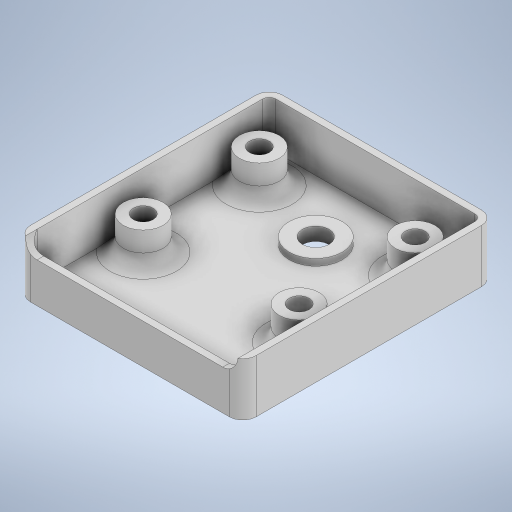
# Autodesk Inventor part: MKSMount
Saved by Autodesk Inventor 2024.2 (Build 282272000, 272)
## iProperties
Created: 2024-06-06
Part Number: MKSMount
Material: Generic
Document SubType Name: Modeling
Designer: Robin
Density: 1 g/cm^3
Appearance: Default
Author: Robin
Autodesk Inventor part; units mm, degrees
ref_plane "YZ Plane" through (0, 0, 0) normal (1, 0, 0) x (0, 1, 0)
ref_plane "XZ Plane" through (0, 0, 0) normal (0, 1, 0) x (-1, 0, 0)
ref_plane "XY Plane" through (0, 0, 0) normal (0, 0, 1) x (1, 0, 0)
sketch "Sketch1" plane through (0, 0, 0) normal (0, 1, 0) x (-1, 0, 0)
  line L0 (17, 19) -> (-17, 19)
  line L1 (-17, 19) -> (-17, -19)
  line L2 (-17, -19) -> (17, -19)
  line L3 (17, -19) -> (17, 19)
  point P0 (0, 0)
  point P1 (0, 19)
  point P2 (17, 0)
  dimension "d0" = 38
  dimension "d1" = 34
  constraints: 8 end point, 2 midpoint, 2 parallel, 1 horizontal, 1 horizontal alignment, 1 perpendicular, 1 vertical alignment
  measures "d0" distance of L2.end L0.start
  measures "d1" distance of L0.start L0.end
extrude "Extrusion1" add sketch "Sketch1" along normal blind 8
shell "Shell1" thickness 1 removed faces 1 at (5.6667, 8, 6.3333)
sketch "Sketch2" plane through (-16, 1, -18) normal (0, 1, 0) x (1, 0, 0)
  circle A0 centre (4, -23) radius 3
  circle A1 centre (4, -5.5) radius 3
  circle A2 centre (27.5, -23) radius 3
  circle A3 centre (27.5, -5.5) radius 3
  line L0 (32, -36) -> (0, -36) projected
  line L1 (0, -36) -> (0, 0) projected
  circle A4 centre (4, -23) radius 1.5
  circle A5 centre (4, -5.5) radius 1.5
  circle A6 centre (27.5, -5.5) radius 1.5
  circle A7 centre (27.5, -23) radius 1.5
  point P0 (16, -18)
  dimension "d7" = 6
  dimension "d8" = 6
  dimension "d9" = 6
  dimension "d10" = 6
  dimension "d11" = 13
  dimension "d12" = 17.5
  dimension "d13" = 4
  dimension "d14" = 23.5
  dimension "d17" = 3
  dimension "d18" = 3
  dimension "d19" = 3
  dimension "d20" = 3
  constraints: 8 centre point, 4 coincident, 2 horizontal alignment, 2 vertical alignment
  measures "d7" diameter of A0
  measures "d8" diameter of A1
  measures "d9" diameter of A2
  measures "d10" diameter of A3
  measures "d11" distance from line of L0 A0.centre
  measures "d12" distance of A1.centre A0.centre
  measures "d13" distance from line of L1 A1.centre
  measures "d14" distance of A2.centre A0.centre
  measures "d17" diameter of A4
  measures "d18" diameter of A5
  measures "d19" diameter of A6
  measures "d20" diameter of A7
extrude "Extrusion2" add sketch "Sketch2" along normal blind 5
fillet "Fillet1" radius 2 4 edges at (8.5, 1, 5) (-15, 1, 5) (-15, 1, -12.5) (8.5, 1, -12.5)
sketch "Sketch3" plane through (-16, 1, -18) normal (0, 1, 0) x (1, 0, 0)
  circle A0 centre (16, -9) radius 2
  line L0 (33, 1) -> (-1, 1) projected
  point P0 (16, -18)
  point P1 (16, 1)
  dimension "d22" = 10
  dimension "d23" = 4
  constraints: 1 centre point, 1 midpoint, 1 vertical alignment
  measures "d22" distance from line of L0 A0.centre
  measures "d23" diameter of A0
extrude "Extrusion3" cut sketch "Sketch3" against normal blind 4
sketch "Sketch4" plane through (-16, 1, -18) normal (0, 1, 0) x (1, 0, 0)
  circle A0 centre (16, -9) radius 2 projected
  circle A1 centre (16, -9) radius 4
  point P0 (16, -18)
  dimension "d26" = 8
  constraints: 1 centre point, 1 coincident
  measures "d26" diameter of A1
extrude "Extrusion4" add sketch "Sketch4" along normal blind 1
sketch "Sketch5" plane through (-17, 0, 19) normal (0, 0, 1) x (1, 0, 0)
  line L0 (1, 6) -> (33, 6)
  line L1 (33, 6) -> (33, 8)
  line L2 (33, 8) -> (1, 8)
  line L3 (1, 8) -> (1, 6)
  line L4 (0, 0) -> (0, 8) projected
  line L5 (34, 0) -> (34, 8) projected
  point P0 (17, 0)
  dimension "d30" = 1
  dimension "d31" = 1
  dimension "d32" = 2
  constraints: 8 end point, 2 parallel, 1 horizontal, 1 horizontal alignment, 1 perpendicular
  measures "d30" distance between parallel lines of L4 L3
  measures "d31" distance between parallel lines of L5 L1
  measures "d32" distance between parallel lines of L2 L0
extrude "Extrusion5" cut sketch "Sketch5" against normal blind 1
fillet "Fillet2" radius 2 2 edges at (-16, 6, 18.5) (16, 6, 18.5)
fillet "Fillet3" radius 2 4 edges at (-17, 4, 19) (-17, 4, -19) (17, 4, 19) (17, 4, -19)
fillet "Fillet4" radius 1 6 edges at (16, 4.5, -18) (-16, 4.5, -18) (-16, 7, 18) (-16, 3.5, 18) (16, 7, 18) (16, 3.5, 18)
body "Solid1"
